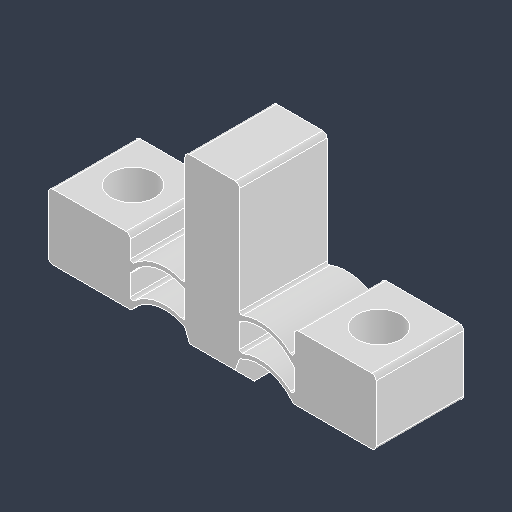
# Autodesk Inventor part: Actuator 2
Saved by Autodesk Inventor 2023.4 (Build 274418000, 418)
## iProperties
Created: 2024-02-27
Part Number: Actuator 2
Material: Generic
Document SubType Name: Modeling
Designer: JoaoSilva
Density: 1 g/cm^3
Appearance: Default
Author: JoaoSilva
Autodesk Inventor part; units mm, degrees
ref_plane "YZ Plane" through (0, 0, 0) normal (1, 0, 0) x (0, 1, 0)
ref_plane "XZ Plane" through (0, 0, 0) normal (0, 1, 0) x (-1, 0, 0)
ref_plane "XY Plane" through (0, 0, 0) normal (0, 0, 1) x (1, 0, 0)
sketch "Sketch1" plane through (0, 0, 0) normal (0, 0, 1) x (1, 0, 0)
  line L0 (-2.5, 9) -> (2.5, 9)
  line L1 (2.5, 9) -> (2.5, -9)
  line L2 (2.5, -9) -> (-2.5, -9)
  line L3 (-2.5, -9) -> (-2.5, 9)
  line L4 (-2.5, 9) -> (2.5, -9) construction
  line L5 (2.5, 9) -> (-2.5, -9) construction
  line L6 (-15, 0) -> (-7.5, 0)
  line L7 (-7.5, 0) -> (-7.5, -3)
  line L8 (-7.5, -3) -> (-15, -3)
  line L9 (-15, -3) -> (-15, 0)
  line L10 (7.5, 0) -> (15, 0)
  line L11 (15, 0) -> (15, -3)
  line L12 (15, -3) -> (7.5, -3)
  line L13 (7.5, -3) -> (7.5, 0)
  line L14 (7.5, -3) -> (7.5, -6)
  line L15 (7.5, -6) -> (15, -6)
  line L16 (15, -6) -> (15, -3)
  line L17 (-7.5, -3) -> (-7.5, -6)
  line L18 (-7.5, -6) -> (-15, -6)
  line L19 (-15, -6) -> (-15, -3)
  line L20 (-7.5, -1.5) -> (7.5, -1.5) construction
  line L21 (-1, -9) -> (-2.5, -4.8788)
  line L22 (1, -9) -> (2.5, -4.8788)
  arc A0 (-2.5, -4.6788) -> (-7.5, -5.8) centre (-4.3279, -8.2367) ccw construction
  arc A1 (-2.4086, -4.5009) -> (-7.6586, -5.6782) centre (-4.3279, -8.2367) ccw
  arc A2 (-2.5914, -4.8567) -> (-7.3414, -5.9218) centre (-4.3279, -8.2367) ccw
  arc A3 (-2.5914, -4.8567) -> (-2.4086, -4.5009) centre (-2.5, -4.6788) ccw
  arc A4 (-7.6586, -5.6782) -> (-7.3414, -5.9218) centre (-7.5, -5.8) ccw
  arc A5 (7.5, -5.8) -> (2.5, -4.6788) centre (4.3279, -8.2367) ccw construction
  arc A6 (7.6586, -5.6782) -> (2.4086, -4.5009) centre (4.3279, -8.2367) ccw
  arc A7 (7.3414, -5.9218) -> (2.5914, -4.8567) centre (4.3279, -8.2367) ccw
  arc A8 (7.3414, -5.9218) -> (7.6586, -5.6782) centre (7.5, -5.8) ccw
  arc A9 (2.4086, -4.5009) -> (2.5914, -4.8567) centre (2.5, -4.6788) ccw
  arc A10 (-2.5, -1.6788) -> (-7.5, -2.8) centre (-4.3279, -5.2367) ccw construction
  arc A11 (-2.4086, -1.5009) -> (-7.6586, -2.6782) centre (-4.3279, -5.2367) ccw
  arc A12 (-2.5914, -1.8567) -> (-7.3414, -2.9218) centre (-4.3279, -5.2367) ccw
  arc A13 (-2.5914, -1.8567) -> (-2.4086, -1.5009) centre (-2.5, -1.6788) ccw
  arc A14 (-7.6586, -2.6782) -> (-7.3414, -2.9218) centre (-7.5, -2.8) ccw
  arc A15 (7.5, -2.8) -> (2.5, -1.6788) centre (4.3279, -5.2367) ccw construction
  arc A16 (7.6586, -2.6782) -> (2.4086, -1.5009) centre (4.3279, -5.2367) ccw
  arc A17 (7.3414, -2.9218) -> (2.5914, -1.8567) centre (4.3279, -5.2367) ccw
  arc A18 (7.3414, -2.9218) -> (7.6586, -2.6782) centre (7.5, -2.8) ccw
  arc A19 (2.4086, -1.5009) -> (2.5914, -1.8567) centre (2.5, -1.6788) ccw
  point P0 (0, 0)
  point P1 (0, -1.5)
  point P2 (-7.5, -5.484)
  point P3 (-2.5, -1.8788)
  point P4 (-2.5, -4.4553)
  point P5 (7.5, -5.484)
  point P6 (2.5, -4.4553)
  point P7 (2.5, -1.8788)
  point P8 (7.5, -2.484)
  point P9 (2.5, -1.4553)
  point P10 (-2.5, -1.4553)
  point P11 (-7.5, -2.484)
  dimension "d0" = 5
  dimension "d1" = 18
  dimension "d2" = 30
  dimension "d3" = 3
  dimension "d4" = 3
  dimension "d5" = 5
  dimension "d8" = 9
  dimension "d9" = 3
  dimension "d10" = 2
  dimension "d11" = 20
  dimension "d12" = 0.4
  dimension "d13" = 4
  dimension "d14" = 3
  constraints: 46 end point, 42 point on circle, 20 centre point, 18 tangent, 14 point on line, 7 perpendicular, 6 equal radius, 6 parallel, 5 midpoint, 3 collinear, 3 equal length, 3 horizontal, 3 vertical alignment, 2 horizontal alignment, 2 vertical
  measures "d0" distance of L0.start L0.end
  measures "d1" distance of L0.end L1.end
  measures "d2" distance between parallel lines of L11 L9
  measures "d3" distance between parallel lines of L2 L18
  measures "d4" distance between parallel lines of L2 L15
  measures "d5" distance between parallel lines of L3 L17
  measures "d8" distance between parallel lines of L2 L6
  measures "d9" distance of L8.end L6.start
  measures "d10" distance of L22.start L21.start
  measures "d11" angle of L3 L21
  measures "d12" radial gap between concentric circles of A1 A2
  measures "d13" radius of A0
  measures "d14" distance of A0.centre A10.centre
extrude "Extrusion1" add sketch "Sketch1" along normal blind 8 contours L0 L1 A16 A19 A6 A9 L22 L2 L21 A3 A1 L3 A13 A11 | A11 A13 L3 | L3 A13 A12 A14 L7 A11 | A16 L13 A18 A17 A19 L1 | L1 A19 A16 | A11 A14 L8 L9 L6 L7 | L7 A14 A11 | A16 A18 L13 | L13 L10 L11 L12 A18 A16 | A1 A3 L3 | L3 A3 A2 A4 L17 A1 | L17 A1 A4 L18 L19 L8 | A6 L14 A8 A7 A9 L1 | L1 A9 A6 | L12 L16 L15 A8 A6 L14 | L17 A4 A1 | A6 A8 L14
chamfer "Chamfer1" distance 3 angle 45 1 edges at (0, -9, 0) measured on face at (0, -9, 0.5)
chamfer "Chamfer2" distance 3 angle 45 1 edges at (0, -9, 8) measured on face at (0, -9, 7.5)
fillet "Fillet1" radius 0.2 14 edges at (-7.5, -2.484, 4) (-7.5, -3, 4) (-7.5, -5.484, 4) (-2.5, -4.8788, 4) (-2.5, -4.4553, 4) (-2.5, -1.8788, 4) (-2.5, -1.4553, 4) (2.5, -1.4553, 4) (2.5, -1.8788, 4) (2.5, -4.4553, 4) (2.5, -4.8788, 4) (7.5, -5.484, 4) (7.5, -3, 4) (7.5, -2.484, 4)
fillet "Fillet2" radius 0.4 10 edges at (-15, 0, 4) (15, 0, 4) (7.5, 0, 4) (15, -6, 4) (-15, -6, 4) (-7.5, 0, 4) (-2.5, 9, 4) (2.5, 9, 4) (-1, -9, 4) (1, -9, 4)
sketch "Sketch3" plane through (-14.6, 0, 0) normal (0, 1, 0) x (1, 0, 0)
  line L0 (3.35, -4) -> (25.85, -4) construction
  line L1 (16.7, 0) -> (12.5, 0) projected
  line L2 (29.2, 0) -> (29.2, -8) projected
  line L3 (6.7, -8) -> (0, -8) projected
  point P0 (14.6, 0)
  point P1 (14.6, -4)
  point P2 (14.6, 0)
  point P3 (29.2, -4)
  point P4 (3.35, -8)
  constraints: 4 midpoint, 2 end point, 2 vertical alignment, 1 horizontal, 1 horizontal alignment
hole "Hole2" at (-11.25, 0, 4) at (11.25, 0, 4) direction (0, -1, 0) diameter 4 end through all
equation "\"d4\" = d3"
body "Solid1"
